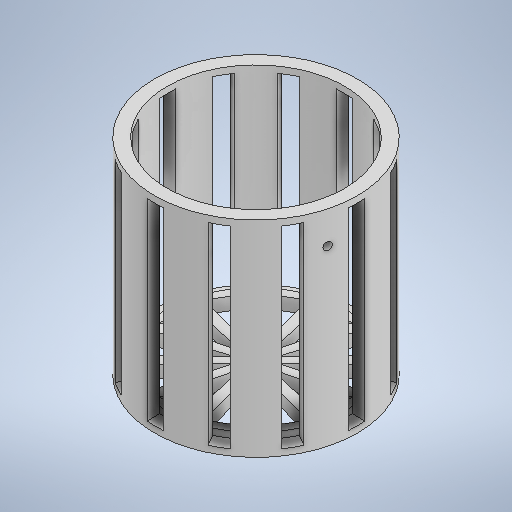
# Autodesk Inventor part: Printable Grate
Saved by Autodesk Inventor 2025 (Build 290162000, 162)
## iProperties
Created: 2024-07-19
Part Number: Printable Grate
Material: Generic
Document SubType Name: Modeling
Designer: track
Density: 1 g/cm^3
Appearance: Default
Author: track
Autodesk Inventor part; units mm, degrees
ref_plane "XZ Plane" through (0, 0, 0) normal (0, 1, 0) x (-1, 0, 0)
ref_plane "XY Plane" through (0, 0, 0) normal (0, 0, 1) x (1, 0, 0)
sketch "Sketch1" plane through (0, 0, 0) normal (0, 1, 0) x (-1, 0, 0)
  circle A0 centre (0, 0) radius 35
  circle A1 centre (0, 0) radius 40
  dimension "d0" = 70
  dimension "d1" = 5
  constraints: 2 centre point, 1 coincident
  measures "d0" diameter of A0
  measures "d1" radial gap between concentric circles of A0 A1
extrude "Extrusion1" add sketch "Sketch1" against normal blind 76.2
sketch "Sketch2" plane through (0, -76.2, 0) normal (0, -1, 0) x (1, 0, 0)
  circle A0 centre (0, 0) radius 40
  circle A1 centre (0, 0) radius 40 projected
  dimension "d4" = 0
  constraints: 1 centre point, 1 coincident
  measures "d4" radial gap between concentric circles of A1 A0
extrude "Extrusion2" add sketch "Sketch2" along normal blind 5
sketch "Sketch3" plane through (0, -81.2, 0) normal (0, -1, 0) x (1, 0, 0)
  line L0 (0, 0) -> (0, 40) construction
  circle A0 centre (0, 0) radius 40 projected
  line L1 (0, 6.35) -> (-6.35, 31.75)
  line L2 (-6.35, 31.75) -> (6.35, 31.75)
  line L3 (6.35, 31.75) -> (0, 6.35)
  dimension "d7" = 12.7
  dimension "d8" = 6.35
  dimension "d9" = 25.4
  constraints: 8 end point, 1 perpendicular, 1 point on line, 1 vertical, 1 vertical alignment, 2 other
  measures "d7" distance of L1.end L2.end
  measures "d8" distance of L0.start L1.start
  measures "d9" distance from line of L2 L1.start
extrude "Extrusion3" cut sketch "Sketch3" against normal up to surface (5 mm away) contours L1 L2 L3
pattern_circular "Circular Pattern1" count 12 over 360 about axis through (0, 0, 0) along (0, -1, 0) of "Extrusion3"
ref_plane "Work Plane1" through (-40, 0, 0) normal (1, 0, 0) x (0, 1, 0)
sketch "Sketch4" plane through (-40, 0, 0) normal (1, 0, 0) x (0, 1, 0)
  line L0 (0, 0) -> (-81.2, 0) construction
  line L1 (-81.2, 40) -> (-81.2, -40) projected
  line L2 (-78.7, -3.175) -> (-2.5, -3.175)
  line L3 (-2.5, -3.175) -> (-2.5, 3.175)
  line L4 (-2.5, 3.175) -> (-78.7, 3.175)
  line L5 (-78.7, 3.175) -> (-78.7, -3.175)
  line L6 (-78.7, -3.175) -> (-2.5, 3.175) construction
  line L7 (-2.5, -3.175) -> (-78.7, 3.175) construction
  point P0 (-40.6, 0)
  dimension "d15" = 76.2
  dimension "d16" = 6.35
  constraints: 14 end point, 4 midpoint, 2 parallel, 1 horizontal, 1 perpendicular
  measures "d15" distance of L3.end L4.end
  measures "d16" distance between parallel lines of L2 L4
extrude "Extrusion4" cut sketch "Sketch4" along normal up to surface round surface about axis through (0, 0, 0) along (0, -1, 0) radius 35 far side no
pattern_circular "Circular Pattern2" count 12 over 360 about axis through (0, 0, 0) along (0, -1, 0) of "Extrusion4"
sketch "Sketch6" plane through (0, 0, 0) normal (0, 1, 0) x (1, 0, 0)
  line L0 (0, 0) -> (38.6368, -10.3536)
  line L1 (5.4993, -3.175) -> (30.6713, -10.3757) projected
  line L2 (31.75, -6.35) -> (6.35, 0) projected
  circle A0 centre (0, 0) radius 40 projected
  dimension "d22" = 1.928
  dimension "d23" = 0.965
  constraints: 2 end point, 2 other
  measures "d22" angle of L1 L2
  measures "d23" angle of L2 L0
ref_plane "Work Plane3" through (38.6368, 0, 10.3536) normal (0.9659202, 0, 0.25884) x (0, 1, 0)
sketch "Sketch7" plane through (38.6368, 0, 10.3536) normal (0.9659202, 0, 0.25884) x (0, 1, 0)
  line L0 (0, 0) -> (-26.9854, 0)
  circle A0 centre (-12.7, 0) radius 1.5
  line L1 (0, -40) -> (0, 40) projected
  dimension "d24" = 3
  dimension "d25" = 12.7
  constraints: 2 end point, 1 centre point, 1 horizontal, 1 point on line
  measures "d24" diameter of A0
  measures "d25" distance from line of L1 A0.centre
extrude "Extrusion5" cut sketch "Sketch7" against normal up to surface round surface about axis through (0, 0, 0) along (0, -1, 0) radius 35 far side no
body "Solid1"
